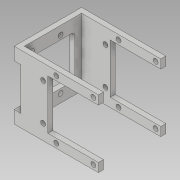
# Autodesk Inventor part: connection_linkFour
Saved by Autodesk Inventor 2017 (Build 210142000, 142)
## iProperties
Part Number: connection_linkFour
Material: Aluminium 6061
Document SubType Name: Modeling
Designer: Max
Density: 2.7 g/cm^3
Appearance: Vorgabe
Mass: 15.4018 g
Surface Area: 53.3174 cm^2
Volume: 5.70436 cm^3
Author: Max
Autodesk Inventor part; units mm, degrees
ref_plane "YZ Plane" through (0, 0, 0) normal (1, 0, 0) x (0, 1, 0)
ref_plane "XZ Plane" through (0, 0, 0) normal (0, 1, 0) x (-1, 0, 0)
ref_plane "XY Plane" through (0, 0, 0) normal (0, 0, 1) x (1, 0, 0)
sketch "Skizze1" plane through (0, 0, 0) normal (1, 0, 0) x (0, 1, 0)
  line L0 (-20, 20) -> (20, 20)
  line L1 (20, 20) -> (20, -20)
  line L2 (20, -20) -> (-20, -20)
  line L3 (-20, -20) -> (-20, 20)
  line L4 (-20, 20) -> (20, -20) construction
  line L5 (20, 20) -> (-20, -20) construction
  point P0 (0, 0)
  dimension "d0" = 40
  dimension "d1" = 40
  constraints: 12 end point, 2 midpoint, 2 parallel, 1 horizontal, 1 perpendicular
  measures "d0" distance of L1.end L2.end
  measures "d1" distance of L0.end L1.end
extrude "Extrusion1" add sketch "Skizze1" along normal blind 50
sketch "Skizze2" plane through (0, -20, 20) normal (0, 0, 1) x (1, 0, 0)
  line L0 (0, 0) -> (0, 40) projected
  line L1 (0, 0) -> (50, 0) projected
  line L2 (50, 40) -> (50, 0) projected
  line L3 (0, 40) -> (50, 40) projected
  line L4 (50, 40) -> (50, 0) projected
  line L5 (50, 37) -> (3, 37)
  line L6 (3, 37) -> (3, 3)
  line L7 (3, 3) -> (50, 3)
  line L8 (50, 3) -> (50, 37)
  point P0 (0, 20)
  dimension "d4" = 3
  dimension "d5" = 3
  dimension "d6" = 3
  constraints: 8 end point, 2 parallel, 1 horizontal, 1 perpendicular, 1 point on line
  measures "d4" distance between parallel lines of L5 L3
  measures "d5" distance between parallel lines of L1 L7
  measures "d6" distance between parallel lines of L0 L6
extrude "Extrusion2" cut sketch "Skizze2" against normal through all contours L7 L6 L5 L2
sketch "Skizze3" plane through (0, -20, -20) normal (0, -1, 0) x (1, 0, 0)
  line L0 (0, 0) -> (0, 40) projected
  line L1 (0, 0) -> (50, 0) projected
  line L2 (50, 40) -> (50, 0) projected
  line L3 (0, 40) -> (50, 40) projected
  line L4 (0, 20) -> (44.7617, 20) construction
  line L5 (20, 34.75) -> (50, 34.75)
  line L6 (50, 34.75) -> (50, 5.25)
  line L7 (50, 5.25) -> (20, 5.25)
  line L8 (20, 5.25) -> (20, 34.75)
  line L9 (20, 34.75) -> (50, 5.25) construction
  line L10 (50, 34.75) -> (20, 5.25) construction
  point P0 (35, 20)
  dimension "d9" = 29.5
  dimension "d10" = 30
  constraints: 14 end point, 2 horizontal, 2 midpoint, 2 parallel, 2 point on line, 1 perpendicular
  measures "d9" distance of L7.end L5.start
  measures "d10" distance of L6.end L7.end
extrude "Extrusion3" cut sketch "Skizze3" against normal blind 40 contours L7 L8 L5 L2
sketch "Skizze4" plane through (0, -20, -20) normal (0, -1, 0) x (1, 0, 0)
  line L0 (50, 5.25) -> (20, 5.25) projected
  line L1 (20, 5.25) -> (20, 34.75) projected
  line L2 (20, 34.75) -> (50, 34.75) projected
  line L3 (50, 40) -> (50, 34.75) projected
  line L4 (0, 40) -> (50, 40) projected
  line L5 (0, 0) -> (0, 40) projected
  line L6 (0, 0) -> (50, 0) projected
  line L7 (50, 5.25) -> (50, 0) projected
  line L8 (0, 20) -> (84.4351, 20) construction
  point P0 (25, 37.3)
  point P1 (25, 2.7)
  point P2 (17.2, 31)
  point P3 (17.2, 9)
  point P4 (47, 37.3)
  point P5 (47, 2.7)
  dimension "d13" = 5
  dimension "d14" = 5
  dimension "d15" = 34.6
  dimension "d16" = 17.3
  dimension "d17" = 22
  dimension "d18" = 11
  dimension "d19" = 2.8
  dimension "d20" = 2.8
  dimension "d47" = 17.3
  dimension "d48" = 17.3
  dimension "d49" = 22
  dimension "d50" = 22
  constraints: 2 end point, 1 horizontal
  measures "d13" distance from line of point (25, 2.7) L1
  measures "d14" distance from line of L1 point (25, 37.3)
  measures "d15" distance of point (25, 2.7) point (25, 37.3)
  measures "d16" distance from line of L8 point (25, 37.3)
  measures "d17" distance of point (17.2, 9) point (17.2, 31)
  measures "d18" distance from line of L8 point (17.2, 31)
  measures "d19" distance from line of L1 point (17.2, 31)
  measures "d20" distance from line of L1 point (17.2, 9)
  measures "d47" distance from line of point (47, 37.3) L8
  measures "d48" distance from line of L8 point (47, 2.7)
  measures "d49" distance of point (47, 37.3) point (25, 37.3)
  measures "d50" distance of point (47, 2.7) point (25, 2.7)
hole "Bohrung1" at (25, -20, 17.3) at (25, -20, -17.3) at (17.2, -20, 11) at (17.2, -20, -11) at (47, -20, 17.3) at (47, -20, -17.3) direction (0, 1, 0) diameter 2.9 end through all clearance for "Inbusschraube ISO 4762" size "M2.5" standard "ISO"
sketch "Skizze5" plane through (0, -20, -20) normal (0, -1, 0) x (1, 0, 0)
  line L0 (-4, 32.5) -> (4, 32.5)
  line L1 (4, 32.5) -> (4, 7.5)
  line L2 (4, 7.5) -> (-4, 7.5)
  line L3 (-4, 7.5) -> (-4, 32.5)
  line L4 (-4, 32.5) -> (4, 7.5) construction
  line L5 (4, 32.5) -> (-4, 7.5) construction
  circle A0 centre (17.2, 31) radius 1.45 projected
  circle A1 centre (25, 37.3) radius 1.45 projected
  circle A2 centre (25, 2.7) radius 1.45 projected
  circle A3 centre (17.2, 9) radius 1.45 projected
  line L6 (50, 5.25) -> (20, 5.25) projected
  line L7 (20, 5.25) -> (20, 34.75) projected
  line L8 (20, 34.75) -> (50, 34.75) projected
  line L9 (50, 40) -> (50, 34.75) projected
  line L10 (0, 40) -> (50, 40) projected
  line L11 (0, 0) -> (0, 40) projected
  line L12 (0, 0) -> (50, 0) projected
  line L13 (50, 5.25) -> (50, 0) projected
  point P0 (0, 20)
  dimension "d28" = 25
  dimension "d30" = 4
  constraints: 12 end point, 2 midpoint, 2 parallel, 1 horizontal, 1 perpendicular
  measures "d28" distance of L2.end L0.start
  measures "d30" distance between parallel lines of L1 L11
extrude "Extrusion4" cut sketch "Skizze5" against normal blind 33 contours L0 L11 L2 L3 | L0 L1 L2 L11
sketch "Skizze6" plane through (0, 0, 0) normal (-1, 0, 0) x (0, 0, 1)
  line L0 (0, -27.3201) -> (0, 32.8288) construction
  line L1 (-15, -12.5) -> (15, -12.5) construction
  line L2 (15, -12.5) -> (15, 4.5) construction
  line L3 (15, 4.5) -> (-15, 4.5) construction
  line L4 (-15, 4.5) -> (-15, -12.5) construction
  line L5 (-15, -12.5) -> (15, 4.5) construction
  line L6 (15, -12.5) -> (-15, 4.5) construction
  point P0 (0, 0)
  point P1 (0, -4)
  dimension "d34" = 17
  dimension "d44" = 4
  dimension "d45" = 30
  constraints: 14 end point, 2 midpoint, 2 parallel, 2 point on line, 1 horizontal, 1 perpendicular, 1 vertical
  measures "d34" distance of L3.end L1.start
  measures "d44" distance of point (0, -4) point (0, 0)
  measures "d45" distance of L1.start L1.end
hole "Bohrung2" at (0, 4.5, -15) at (0, -12.5, -15) at (0, 4.5, 15) at (0, -12.5, 15) direction (1, 0, 0) diameter 2.9 end through all clearance for "Inbusschraube ISO 4762" size "M2.5" standard "ISO"
fillet "Rundung1" radius 2 2 edges at (1.5, 13, 12.5) (1.5, 13, -12.5)
equation "\"d5\" = d4"
equation "\"d13\" = d14"
equation "\"d16\" = 0.5 * d15"
equation "\"d18\" = 0.5 * d17"
equation "\"d20\" = d19"
equation "\"d47\" = d16"
equation "\"d48\" = d16"
equation "\"d50\" = d49"
